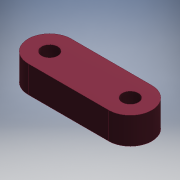
# Autodesk Inventor part: Link_VAM
Saved by Autodesk Inventor 2016 (Build 200138000, 138)
## iProperties
Created: 2015-12-07
Part Number: Link_VAM
Material: Generic
Document SubType Name: Modeling
Designer: lk8187
Density: 1 g/cm^3
Appearance: Smooth - Dark Maroon
Author: lk8187
Autodesk Inventor part; units mm, degrees
ref_plane "YZ Plane" through (0, 0, 0) normal (1, 0, 0) x (0, 1, 0)
ref_plane "XZ Plane" through (0, 0, 0) normal (0, 1, 0) x (-1, 0, 0)
ref_plane "XY Plane" through (0, 0, 0) normal (0, 0, 1) x (1, 0, 0)
sketch "Sketch1" plane through (0, 0, 0) normal (0, 0, 1) x (1, 0, 0)
  line L0 (0, 0) -> (15, 0) construction
  line L1 (0, -4) -> (15, -4)
  line L2 (15, 4) -> (0, 4)
  arc A0 (0, 4) -> (0, -4) centre (0, 0) ccw
  arc A1 (15, -4) -> (15, 4) centre (15, 0) ccw
  circle A2 centre (0, 0) radius 1.5
  circle A3 centre (15, 0) radius 1.5
  point P0 (7.5, 0)
  dimension "d0" = 15
  dimension "d1" = 3
  dimension "d2" = 8
  constraints: 8 end point, 4 centre point, 4 point on circle, 4 tangent, 2 coincident, 1 equal radius, 1 horizontal, 1 midpoint, 1 parallel
  measures "d0" distance of L0.start L0.end
  measures "d1" diameter of A2
  measures "d2" distance between parallel lines of L1 L2
extrude "Extrusion1" add sketch "Sketch1" along normal blind 5
body "Solid1"
